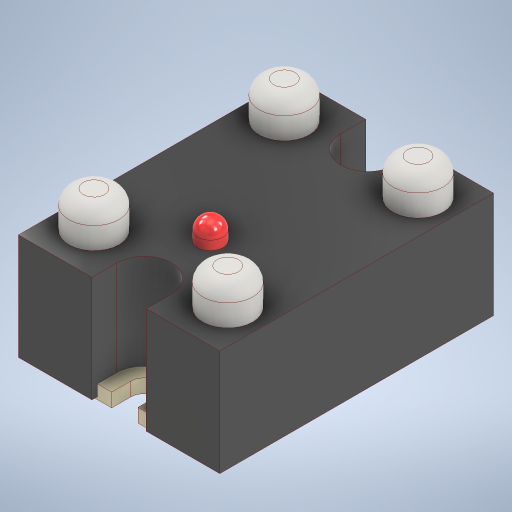
# Autodesk Inventor part: solid state relay
Saved by Autodesk Inventor 2023 (Build 270158030, 158C)
## iProperties
Created: 2024-03-26
Part Number: solid state relay
Material: Generic
Document SubType Name: Modeling
Designer: Imogen Heard
Density: 1 g/cm^3
Appearance: Light Red
Author: Imogen Heard
Autodesk Inventor part; units mm, degrees
ref_plane "YZ Plane" through (0, 0, 0) normal (1, 0, 0) x (0, 1, 0)
ref_plane "XZ Plane" through (0, 0, 0) normal (0, 1, 0) x (-1, 0, 0)
sketch "Sketch1" plane through (0, 0, 0) normal (0, 1, 0) x (-1, 0, 0)
  line L0 (13.1, -18.1) -> (-13.1, -18.1)
  line L1 (-13.1, -18.1) -> (-13.1, 18.1)
  line L2 (13.1, 18.1) -> (13.1, -18.1)
  circle A0 centre (0, -15.45) radius 1.82
  arc A1 (-1.82, 15.45) -> (1.82, 15.45) centre (0, 15.45) ccw
  line L3 (-1.82, 15.45) -> (-1.82, 18.1)
  line L4 (1.82, 15.45) -> (1.82, 18.1)
  line L5 (-13.1, 18.1) -> (-1.82, 18.1)
  line L6 (1.82, 18.1) -> (13.1, 18.1)
  point P0 (0, 0)
  dimension "d1" = 26.2
  dimension "d2" = 13.1
  dimension "d6" = 3.64
  dimension "d7" = 2.65
  dimension "d8" = 3.64
  dimension "d10" = 36.2
  dimension "d11" = 18.1
  dimension "d12" = 2.65
  constraints: 14 end point, 5 perpendicular, 3 parallel, 2 centre point, 2 horizontal alignment, 2 point on circle, 2 vertical alignment, 1 horizontal, 1 tangent
  measures "d1" distance between parallel lines of L1 L2
  measures "d2" distance from line of L2 point (0, 0)
  measures "d6" diameter of A0
  measures "d7" distance from line of L0 A0.centre
  measures "d8" diameter of A1
  measures "d10" distance between parallel lines of L0 L6
  measures "d11" distance from line of L6 point (0, 0)
  measures "d12" distance from line of L5 A1.centre
extrude "Extrusion1" add sketch "Sketch1" along normal blind 1.9
ref_plane "Work Plane1" through (0, 0.4, 0) normal (0, -1, 0) x (1, 0, 0)
sketch "Sketch2" plane through (0, 0.4, 0) normal (0, -1, 0) x (1, 0, 0)
  line L0 (1.82, 18.1) -> (13.1, 18.1) projected
  line L1 (13.1, 18.1) -> (13.1, -18.1) projected
  line L2 (13.1, -18.1) -> (-13.1, -18.1) projected
  line L3 (-13.1, -18.1) -> (-13.1, 18.1) projected
  line L4 (-13.1, 18.1) -> (-1.82, 18.1) projected
  line L5 (-1.82, 18.1) -> (-1.82, 15.45) projected
  arc A0 (-1.82, 15.45) -> (1.82, 15.45) centre (0, 15.45) ccw projected
  line L6 (1.82, 15.45) -> (1.82, 18.1) projected
  circle A1 centre (0, -15.45) radius 1.82 projected
  line L7 (-13.9, 18.9) -> (-13.9, -18.9)
  line L8 (13.9, -18.9) -> (13.9, 18.9)
  line L9 (13.9, 18.9) -> (3.75, 18.9)
  line L10 (-3.75, 18.9) -> (-13.9, 18.9)
  line L11 (3.75, 18.9) -> (3.75, 15.45)
  line L12 (-3.75, 15.45) -> (-3.75, 18.9)
  arc A2 (-3.75, 15.45) -> (3.75, 15.45) centre (0, 15.45) ccw
  line L13 (-3.8538, -18.9) -> (-3.75, -18.9)
  line L14 (-13.9, -18.9) -> (-3.8538, -18.9)
  line L15 (3.75, -15.45) -> (3.75, -18.9)
  line L16 (-3.75, -18.9) -> (-3.75, -15.45)
  arc A3 (3.75, -15.45) -> (-3.75, -15.45) centre (0, -15.45) ccw
  line L17 (3.75, -18.9) -> (13.9, -18.9)
  point P0 (0, 0)
  point P1 (-3.75, 45.4974)
  point P2 (-3.8019, -18.9)
  point P3 (3.75, 18.1)
  point P4 (-3.75, 18.1)
  point P5 (-3.75, -18.1)
  point P6 (3.75, -18.1)
  dimension "d14" = 0.8
  dimension "d15" = 7.5
  dimension "d17" = 0.8
  dimension "d18" = 0.8
  dimension "d20" = 0.8
  dimension "d21" = 3.75
  constraints: 22 end point, 10 horizontal alignment, 4 point on circle, 4 vertical alignment, 2 centre point, 2 coincident, 2 parallel, 1 horizontal, 1 midpoint, 1 perpendicular, 1 point on line
  measures "d14" distance between parallel lines of L3 L7
  measures "d15" distance between parallel lines of L11 L12
  measures "d17" distance between parallel lines of L10 L4
  measures "d18" distance between parallel lines of L8 L1
  measures "d20" distance between parallel lines of L14 L2
  measures "d21" radius of A2
extrude "Extrusion2" add sketch "Sketch2" against normal blind 14.66 separate body contours L11 L9 L8 L17 L15 L2 L1 L0 | L0 L1 L2 L15 A3 L16 L3 L4 L12 A2 L11 | L4 L3 L2 L16 L13 L14 L7 L10 L12
sketch "Sketch3" plane through (0, 15.06, 0) normal (0, 1, 0) x (1, 0, 0)
  circle A0 centre (-9.24, 13.14) radius 3.47
  circle A1 centre (9.24, 13.14) radius 3.47
  circle A2 centre (9.24, -13.14) radius 3.47
  circle A3 centre (-9.24, -13.14) radius 3.47
  line L0 (13.9, -18.9) -> (13.9, 18.9) projected
  line L1 (13.9, 18.9) -> (3.75, 18.9) projected
  line L2 (-13.9, 18.9) -> (-13.9, -18.9) projected
  line L3 (3.75, -18.9) -> (13.9, -18.9) projected
  point P0 (0, 0)
  dimension "d26" = 4.66
  dimension "d27" = 5.76
  dimension "d28" = 6.94
  dimension "d29" = 4.66
  dimension "d30" = 5.76
  constraints: 4 centre point, 3 equal radius, 2 horizontal alignment, 2 vertical alignment
  measures "d26" distance from line of A1.centre L0
  measures "d27" distance from line of A1.centre L1
  measures "d28" diameter of A1
  measures "d29" distance from line of L2 A0.centre
  measures "d30" distance from line of L3 A2.centre
extrude "Extrusion3" add sketch "Sketch3" along normal blind 5 separate body
fillet "Fillet1" radius 2 4 edges at (-12.71, 20.06, -13.14) (5.77, 20.06, -13.14) (5.77, 20.06, 13.14) (-12.71, 20.06, 13.14)
sketch "Sketch4" plane through (0, 15.06, 0) normal (0, 1, 0) x (1, 0, 0)
  circle A0 centre (0, -6.3) radius 1.75
  line L0 (3.75, -18.9) -> (13.9, -18.9) projected
  point P0 (0, 0)
  dimension "d34" = 3.5
  dimension "d35" = 12.6
  constraints: 1 centre point, 1 vertical alignment
  measures "d34" diameter of A0
  measures "d35" distance from line of L0 A0.centre
extrude "Extrusion4" add sketch "Sketch4" along normal blind 3 separate body
fillet "Fillet2" radius 1.75 1 edges at (-1.75, 18.06, 6.3)
equation "\"d2\" = 0.5 * d1"
equation "\"d8\" = d6"
equation "\"d12\" = d7"
equation "\"d17\" = d14"
equation "\"d18\" = d17"
equation "\"d29\" = d26"
equation "\"d30\" = d27"
equation "\"d3\" = 0.5 * d0"
equation "\"d9\" = d7"
equation "\"d0\" = 36.2"
